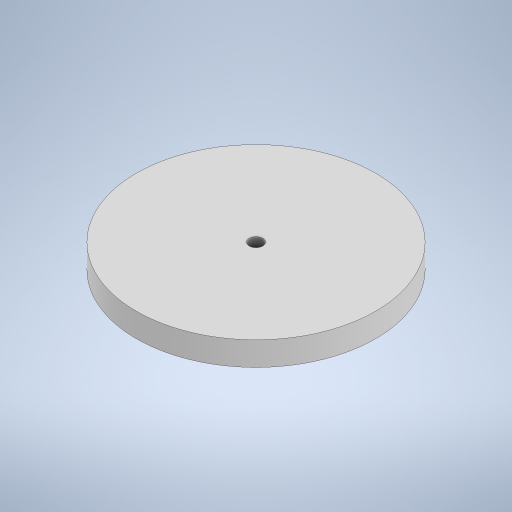
# Autodesk Inventor part: Piston Head
Saved by Autodesk Inventor 2023 (Build 270158030, 158C)
## iProperties
Created: 2022-09-17
Part Number: Piston Head
Material: Generic
Document SubType Name: Modeling
Designer: cjj5381
Density: 1 g/cm^3
Appearance: Default
Author: cjj5381
Autodesk Inventor part; units mm, degrees
ref_plane "YZ Plane" through (0, 0, 0) normal (1, 0, 0) x (0, 1, 0)
ref_plane "XZ Plane" through (0, 0, 0) normal (0, 1, 0) x (-1, 0, 0)
ref_plane "XY Plane" through (0, 0, 0) normal (0, 0, 1) x (1, 0, 0)
sketch "Sketch1" plane through (0, 0, 0) normal (0, 1, 0) x (-1, 0, 0)
  circle A0 centre (0, 0) radius 63.5
  dimension "d0" = 127
  constraints: 1 centre point, 1 coincident
  measures "d0" diameter of A0
extrude "Extrusion1" add sketch "Sketch1" along normal blind 12.7
sketch "Sketch2" plane through (0, 12.7, 0) normal (0, 1, 0) x (1, 0, 0)
  point P0 (0, 0)
  point P1 (26.4475, 5.8254)
hole "Hole1" at (0, 12.7, 0) direction (0, -1, 0) diameter 7.1374 end through all clearance for "Hex Head Bolt" size "1/4" standard "Ansi Unified Screw Threads"
sketch "Sketch3" plane through (0, 0, 0) normal (0, -1, 0) x (1, 0, 0)
  circle A0 centre (0, 0) radius 3.5687 projected
  line L0 (6.4231, 0) -> (3.2116, -5.5626)
  line L1 (3.2116, -5.5626) -> (-3.2116, -5.5626)
  line L2 (-3.2116, -5.5626) -> (-6.4231, 0)
  line L3 (-6.4231, 0) -> (-3.2116, 5.5626)
  line L4 (-3.2116, 5.5626) -> (3.2116, 5.5626)
  line L5 (3.2116, 5.5626) -> (6.4231, 0)
  dimension "d10" = 11.1252
  constraints: 12 end point, 1 coincident, 13 other
  measures "d10" distance between parallel lines of L1 L4
extrude "Extrusion2" cut sketch "Sketch3" against normal blind 4.3688 contours A0 | L0 L1 L2 L3 L4 L5
chamfer "Chamfer1" distance 0.508 angle 45 6 edges at (4.8174, 0, 2.7813) (0, 0, 5.5626) (-4.8174, 0, 2.7813) (-4.8174, 0, -2.7813) (0, 0, -5.5626) (4.8174, 0, -2.7813)
body "Solid1"
